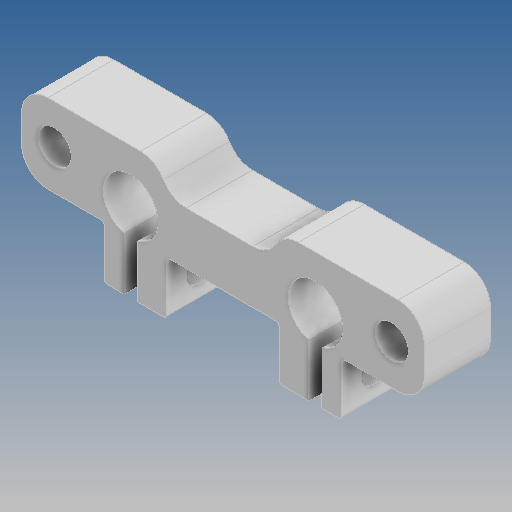
# Autodesk Inventor part: 0008-30-006
Saved by Autodesk Inventor 2020 (Build 240168000, 168)
## iProperties
Created: 2021-05-22
Part Number: 0008-30-006
Material: Generic
Document SubType Name: Modeling
Designer: Iulian Bors
Density: 1 g/cm^3
Appearance: Default
Author: Iulian Bors
Subject: 006
Autodesk Inventor part; units mm, degrees
ref_plane "YZ Plane" through (0, 0, 0) normal (1, 0, 0) x (0, 1, 0)
ref_plane "XZ Plane" through (0, 0, 0) normal (0, 1, 0) x (-1, 0, 0)
ref_plane "XY Plane" through (0, 0, 0) normal (0, 0, 1) x (1, 0, 0)
sketch "Sketch1" plane through (0, 0, 0) normal (0, 0, 1) x (1, 0, 0)
  line L0 (-20.5422, 8) -> (20.5422, 8)
  line L1 (20.5422, 8) -> (20.5422, -12)
  line L2 (20.5422, -12) -> (-20.5422, -12)
  line L3 (-20.5422, -12) -> (-20.5422, 8)
  arc A0 (-13, -4.0277) -> (-15, -4.0277) centre (-14, 0) ccw
  arc A1 (15, -4.0277) -> (13, -4.0277) centre (14, 0) ccw
  line L4 (0, 8) -> (0, -12) construction
  line L5 (-13, -4.0277) -> (-13, -12)
  line L6 (-13, -12) -> (-15, -12)
  line L7 (-15, -12) -> (-15, -4.0277)
  line L8 (15, -4.0277) -> (15, -12)
  line L9 (15, -12) -> (13, -12)
  line L10 (13, -12) -> (13, -4.0277)
  line L11 (-20.5422, -4) -> (-18, -4)
  line L12 (-18, -4) -> (-18, -12)
  line L13 (-18, -12) -> (-20.5422, -12)
  line L14 (-20.5422, -12) -> (-20.5422, -4)
  line L15 (18, -4) -> (20.5422, -4)
  line L16 (20.5422, -4) -> (20.5422, -12)
  line L17 (20.5422, -12) -> (18, -12)
  line L18 (18, -12) -> (18, -4)
  line L19 (-8.5, -4) -> (8.5, -4)
  line L20 (8.5, -4) -> (8.5, -12)
  line L21 (8.5, -12) -> (-8.5, -12)
  line L22 (-8.5, -12) -> (-8.5, -4)
  line L23 (-8.5, 8) -> (8.5, 8)
  line L24 (8.5, 8) -> (8.5, 4)
  line L25 (8.5, 4) -> (-8.5, 4)
  line L26 (-8.5, 4) -> (-8.5, 8)
  point P0 (0, 0)
  point P1 (0, -2)
  point P2 (-14, -4.3116)
  point P3 (14, -4.0277)
  point P4 (0, -4)
  point P5 (-13, -12)
  point P6 (-8.5, -12)
  point P7 (8.5, -12)
  point P8 (20.5422, -4)
  point P9 (8.5, 8)
  point P10 (-8.5, 8)
  point P11 (-15, -12)
  dimension "d0" = 8.3
  dimension "d1" = 28
  dimension "d2" = 2
  dimension "d4" = 2
  dimension "d6" = 41.0844
  dimension "d7" = 8
  dimension "d8" = 12
  dimension "d9" = 20
  dimension "d10" = 3
  dimension "d11" = 3
  dimension "d13" = 8
  dimension "d15" = 5.5
  dimension "d16" = 5.5
  dimension "d17" = 4
  dimension "d18" = 4
  constraints: 54 end point, 12 parallel, 6 collinear, 6 perpendicular, 5 horizontal, 5 midpoint, 4 point on circle, 4 vertical alignment, 3 equal length, 2 centre point, 2 point on line, 1 coincident, 1 equal radius, 1 horizontal alignment, 1 other
  measures "d0" diameter of A0
  measures "d1" distance of A1.centre A0.centre
  measures "d2" distance between parallel lines of L5 L7
  measures "d4" distance between parallel lines of L8 L10
  measures "d6" distance of L0.start L0.end
  measures "d7" distance of L11.end L12.end
  measures "d8" distance from line of L2 A0.centre
  measures "d9" distance of L2.end L0.start
  measures "d10" distance between parallel lines of L7 L12
  measures "d11" distance from line of L18 L8.end
  measures "d13" distance of L17.end L15.start
  measures "d15" distance from line of A0.centre L26
  measures "d16" distance from line of A0.centre L22
  measures "d17" distance from line of L19 point (0, 0)
  measures "d18" distance from line of point (0, 0) L25
extrude "Extrusion1" add sketch "Sketch1" along normal blind 10 contours L0 L26 L25 L24 L1 L15 L18 L2 L8 A1 L10 L20 L19 L22 L5 A0 L7 L12 L11 L3
sketch "Sketch2" plane through (-18, -12, 0) normal (-1, 0, 0) x (0, 0, 1)
  circle A0 centre (5, 4) radius 1.75
  line L0 (0, 0) -> (10, 0) projected
  line L1 (10, 8) -> (10, 0) projected
  circle A1 centre (5, 4) radius 3 construction
  point P0 (0, 12)
  point P1 (5, 0)
  point P2 (10, 4)
  dimension "d22" = 3.5
  dimension "d23" = 6
  constraints: 2 centre point, 2 midpoint, 1 coincident, 1 horizontal alignment, 1 vertical alignment
  measures "d22" diameter of A0
  measures "d23" diameter of A1
hole "Hole1" at (-18, -8, 5) direction (1, 0, 0) diameter 4 end through all
fillet "Fillet2" radius 0.5 8 edges at (-18, -4, 5) (-8.5, -4, 5) (8.5, -4, 5) (18, -4, 5) (-18, -12, 5) (-8.5, -12, 5) (8.5, -12, 5) (18, -12, 5)
sketch "Sketch4" plane through (0, 0, 10) normal (0, 0, 1) x (1, 0, 0)
  line L0 (-30.5422, 8) -> (-20.5422, 8)
  line L1 (-20.5422, 8) -> (-20.5422, -4)
  line L2 (-20.5422, -4) -> (-30.5422, -4)
  line L3 (-30.5422, -4) -> (-30.5422, 8)
  line L4 (20.5422, 8) -> (30.5422, 8)
  line L5 (30.5422, 8) -> (30.5422, -4)
  line L6 (30.5422, -4) -> (20.5422, -4)
  line L7 (20.5422, -4) -> (20.5422, 8)
  line L8 (20.5422, -4) -> (20.5422, 8) projected
  line L9 (18.5, -4) -> (20.5422, -4) projected
  line L10 (20.5422, 8) -> (8.5, 8) projected
  line L11 (-8.5, 8) -> (-20.5422, 8) projected
  line L12 (-20.5422, -4) -> (-18.5, -4) projected
  line L13 (-20.5422, 8) -> (-20.5422, -4) projected
  circle A0 centre (-25.5422, 2) radius 2.5
  circle A1 centre (25.5422, 2) radius 2.5
  point P0 (0, 0)
  point P1 (25.5422, 8)
  point P2 (30.5422, 2)
  point P3 (-30.5422, 2)
  point P4 (-25.5422, 8)
  dimension "d32" = 10
  dimension "d33" = 5
  dimension "d34" = 0
  dimension "d35" = 0
  dimension "d36" = 0
  dimension "d37" = 0
  constraints: 16 end point, 4 midpoint, 4 parallel, 3 collinear, 2 centre point, 2 horizontal, 2 horizontal alignment, 2 perpendicular, 2 vertical alignment, 1 equal radius
  measures "d32" distance of L0.start L0.end
  measures "d33" diameter of A0
  measures "d34" distance between parallel lines of L11 L0
  measures "d35" distance between parallel lines of L12 L2
  measures "d36" distance between parallel lines of L10 L4
  measures "d37" distance between parallel lines of L9 L6
extrude "Extrusion2" add sketch "Sketch4" against normal up to surface (10 mm away)
fillet "Fillet3" radius 4 8 edges at (8.5, 8, 5) (30.5422, 8, 5) (30.5422, -4, 5) (8.5, 4, 5) (-8.5, 4, 5) (-8.5, 8, 5) (-30.5422, 8, 5) (-30.5422, -4, 5)
equation "\"d4\" = d2"
equation "\"d11\" = d10"
equation "\"d13\" = d7"
body "Solid1"
